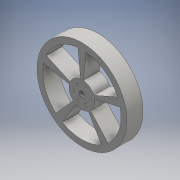
# Autodesk Inventor part: Rueda
Saved by Autodesk Inventor 2016 (Build 200138000, 138)
## iProperties
Created: 2019-03-15
Part Number: Rueda
Material: Genérico
Document SubType Name: Modeling
Designer: FIMCP
Density: 1 g/cm^3
Appearance: Valor por defecto
Author: FIMCP
Autodesk Inventor part; units mm, degrees
ref_plane "YZ Plane" through (0, 0, 0) normal (1, 0, 0) x (0, 1, 0)
ref_plane "XZ Plane" through (0, 0, 0) normal (0, 1, 0) x (-1, 0, 0)
ref_plane "XY Plane" through (0, 0, 0) normal (0, 0, 1) x (1, 0, 0)
sketch "Boceto2" plane through (0, 0, 0) normal (0, 1, 0) x (-1, 0, 0)
  circle A0 centre (0, 0) radius 22.5
  dimension "d8" = 45
  constraints: 1 centre point, 1 coincident
  measures "d8" diameter of A0
extrude "Extrusión1" add sketch "Boceto2" along normal blind 8
sketch "Boceto4" plane through (0, 0, 0) normal (0, 1, 0) x (-1, 0, 0)
  arc A0 (1.118, -1) -> (-1.118, -1) centre (0, 0) ccw
  line L0 (-3.3447, -2.294) -> (-3.3447, -1)
  line L1 (-1.118, -1) -> (1.118, -1)
  dimension "d24" = 3
  dimension "d25" = 1
  constraints: 4 end point, 2 point on circle, 1 centre point, 1 coincident
  measures "d24" diameter of A0
  measures "d25" distance from line of point (0, 0) L1
extrude "Extrusión3" cut sketch "Boceto4" along normal blind 8
sketch "Boceto5" plane through (0, 0, 0) normal (0, 1, 0) x (-1, 0, 0)
  circle A0 centre (-4, 0) radius 0.5
  point P0 (0, 0)
  dimension "d28" = 1
  dimension "d29" = 4
  constraints: 1 centre point
  measures "d28" diameter of A0
  measures "d29" distance of point (0, 0) A0.centre
extrude "Extrusión4" cut sketch "Boceto5" along normal blind 8
pattern_circular "Patrón circular2" count 6 over 360 about axis through (0, -10, 0) along (0, 1, 0) of "Extrusión4"
sketch "Boceto7" plane through (0, 0, 0) normal (0, 1, 0) x (-1, 0, 0)
  arc A0 (-3.25, -5.6292) -> (3.25, -5.6292) centre (0, 0) ccw
  arc A1 (-9.75, -16.8875) -> (9.75, -16.8875) centre (0, 0) ccw
  line L0 (-3.25, -5.6292) -> (-9.75, -16.8875)
  line L1 (0, 0) -> (19.5, 0) construction
  line L2 (3.25, -5.6292) -> (9.75, -16.8875)
  line L3 (0, 0) -> (19.5, 0) construction
  dimension "d37" = 13
  dimension "d38" = 39
  dimension "d39" = 120
  dimension "d40" = 60
  constraints: 8 end point, 4 point on circle, 2 centre point, 2 coincident, 2 horizontal
  measures "d37" diameter of A0
  measures "d38" diameter of A1
  measures "d39" angle of L0 L1
  measures "d40" angle of L2 L3
extrude "Extrusión5" cut sketch "Boceto7" along normal blind 8
pattern_circular "Patrón circular3" count 5 over 360 about axis through (0, -10, 0) along (0, 1, 0) of "Extrusión5"
